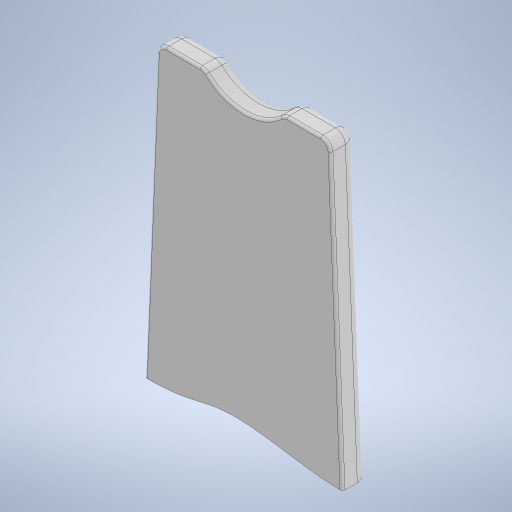
# Autodesk Inventor part: backrest wheelchair EG26
Saved by Autodesk Inventor 2023 (Build 270158000, 158)
## iProperties
Created: 2023-10-18
Part Number: backrest wheelchair EG26
Material: Generic
Document SubType Name: Modeling
Designer: user
Density: 1 g/cm^3
Appearance: Default
Author: user
Autodesk Inventor part; units mm, degrees
ref_plane "YZ Plane" through (0, 0, 0) normal (1, 0, 0) x (0, 1, 0)
ref_plane "XZ Plane" through (0, 0, 0) normal (0, 1, 0) x (-1, 0, 0)
ref_plane "XY Plane" through (0, 0, 0) normal (0, 0, 1) x (1, 0, 0)
sketch "Sketch1" plane through (0, 0, 0) normal (0, 0, 1) x (1, 0, 0)
  line L0 (0, 0) -> (25, 600)
  line L1 (25, 600) -> (375, 600)
  line L2 (375, 600) -> (400, 0)
  line L3 (400, 0) -> (0, 0)
  line L4 (0, 0) -> (76.2678, 0) construction
  line L5 (76.2678, 0) -> (120.3096, 19.0389) construction
  line L6 (120.3096, 19.0389) -> (188.6298, 38.3438) construction
  line L7 (188.6298, 38.3438) -> (327.7567, 0) construction
  line L8 (327.7567, 0) -> (400, 0) construction
  spline S0 degree 4 poles (0, 0) (76.2678, 0) (120.3096, 19.0389) (188.6298, 38.3438) (327.7567, 0) (400, 0) knots 1 1 1 1 1 2 3 3 3 3 3
  arc A0 (120.3096, 600) -> (279.6904, 600) centre (200, 673.1568) ccw
  line L9 (120.3096, 600) -> (25, 600)
  line L10 (25, 600) -> (0, 0)
  dimension "d0" = 600
  dimension "d1" = 25
  dimension "d2" = 350
  dimension "d3" = 400
  dimension "d4" = 175
  constraints: 12 end point, 4 point on line, 2 collinear, 2 point on circle, 1 centre point, 1 horizontal, 1 parallel, 3 other
  measures "d0" vertical distance of L0.start L0.end
  measures "d1" horizontal distance of L0.start L0.end
  measures "d2" distance of L0.end L1.end
  measures "d3" distance of L2.end L0.start
  measures "d4" horizontal distance of L1.end A0.centre
extrude "Extrusion1" add sketch "Sketch1" along normal blind 50 contours L0 L1 A0 L2 S0
fillet "Fillet1" radius 20 9 edges at (327.3452, 600, 0) (387.5, 300, 0) (200, 564.9788, 0) (72.6548, 600, 0) (12.5, 300, 0) (25, 600, 25) (120.3096, 600, 25) (279.6904, 600, 25) (375, 600, 25)
fillet "Fillet2" radius 5 9 edges at (78.071, 600, 50) (119.3501, 598.5837, 50) (200, 564.9788, 50) (280.6499, 598.5837, 50) (321.929, 600, 50) (369.6606, 594.4335, 50) (387.8993, 290.4163, 50) (12.1007, 290.4163, 50) (30.3394, 594.4335, 50)
body "Solid1"
